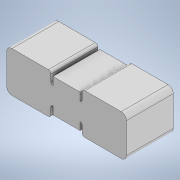
# Autodesk Inventor part: Automoblox Connector
Saved by Autodesk Inventor 2020 (Build 240168000, 168)
## iProperties
Created: 2020-02-04
Part Number: Automoblox Connector
Material: Generic
Document SubType Name: Modeling
Designer: cks4a449
Density: 1 g/cm^3
Appearance: Default
Author: cks4a449
Autodesk Inventor part; units mm, degrees
ref_plane "YZ Plane" through (0, 0, 0) normal (1, 0, 0) x (0, 1, 0)
ref_plane "XZ Plane" through (0, 0, 0) normal (0, 1, 0) x (-1, 0, 0)
ref_plane "XY Plane" through (0, 0, 0) normal (0, 0, 1) x (1, 0, 0)
sketch "Sketch1" plane through (0, 0, 0) normal (0, 0, 1) x (1, 0, 0)
  line L0 (20.32, 9.906) -> (2.54, 9.906)
  line L1 (0, 7.366) -> (0, 0)
  line L2 (22.606, 4.318) -> (22.606, 8.128)
  line L3 (22.606, 8.128) -> (29.21, 8.128)
  line L4 (21.59, 8.636) -> (21.59, 5.334)
  arc A0 (21.59, 5.334) -> (22.606, 4.318) centre (22.606, 5.334) ccw
  arc A1 (2.54, 9.906) -> (0, 7.366) centre (2.54, 7.366) ccw
  arc A2 (21.59, 8.636) -> (20.32, 9.906) centre (20.32, 8.636) ccw
  line L5 (0, 0) -> (29.21, 0) construction
  line L6 (29.21, 0) -> (29.21, 8.128) construction
  line L7 (38.1, 9.906) -> (55.88, 9.906)
  line L8 (58.42, 7.366) -> (58.42, 0)
  line L9 (35.814, 4.318) -> (35.814, 8.128)
  line L10 (35.814, 8.128) -> (29.21, 8.128)
  line L11 (36.83, 8.636) -> (36.83, 5.334)
  arc A3 (35.814, 4.318) -> (36.83, 5.334) centre (35.814, 5.334) ccw
  arc A4 (58.42, 7.366) -> (55.88, 9.906) centre (55.88, 7.366) ccw
  arc A5 (38.1, 9.906) -> (36.83, 8.636) centre (38.1, 8.636) ccw
  line L12 (20.32, -9.906) -> (2.54, -9.906)
  line L13 (0, -7.366) -> (0, 0)
  line L14 (22.606, -4.318) -> (22.606, -8.128)
  line L15 (22.606, -8.128) -> (29.21, -8.128)
  line L16 (21.59, -8.636) -> (21.59, -5.334)
  arc A6 (22.606, -4.318) -> (21.59, -5.334) centre (22.606, -5.334) ccw
  arc A7 (0, -7.366) -> (2.54, -9.906) centre (2.54, -7.366) ccw
  arc A8 (20.32, -9.906) -> (21.59, -8.636) centre (20.32, -8.636) ccw
  line L17 (29.21, 0) -> (29.21, -8.128) construction
  line L18 (38.1, -9.906) -> (55.88, -9.906)
  line L19 (36.83, -8.636) -> (36.83, -5.334)
  arc A9 (55.88, -9.906) -> (58.42, -7.366) centre (55.88, -7.366) ccw
  arc A10 (36.83, -8.636) -> (38.1, -9.906) centre (38.1, -8.636) ccw
  line L20 (35.814, -8.128) -> (29.21, -8.128)
  line L21 (35.814, -4.318) -> (35.814, -8.128)
  arc A11 (36.83, -5.334) -> (35.814, -4.318) centre (35.814, -5.334) ccw
  line L22 (58.42, -7.366) -> (58.42, 0)
  point P0 (0, 9.906)
  point P1 (58.42, 9.906)
  point P2 (0, -9.906)
  point P3 (58.42, -9.906)
  dimension "d7" = 1.016
  dimension "d8" = 5.588
  dimension "d9" = 9.906
  dimension "d10" = 2.54
  dimension "d11" = 1.27
  dimension "d12" = 8.128
  dimension "d13" = 29.21
  constraints: 46 end point, 35 symmetric about line, 24 point on circle, 12 centre point, 8 point on line, 5 tangent, 1 horizontal, 1 line through centre, 1 perpendicular, 1 vertical, 9 other
  measures "d7" distance between parallel lines of L2 L4
  measures "d8" distance from line of L2.start L0
  measures "d9" distance of point (0, 9.906) L1.end
  measures "d10" radius of A1
  measures "d11" radius of A2
  measures "d12" vertical distance of L1.end L3.end
  measures "d13" distance from line of L3.end L1
extrude "Extrusion1" add sketch "Sketch1" along normal blind 22.86
body "Solid1"
